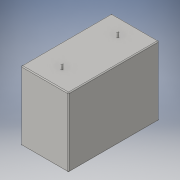
# Autodesk Inventor part: Deep Cycle Battery
Saved by Autodesk Inventor 2016 (Build 200138000, 138)
## iProperties
Created: 2018-07-06
Part Number: Deep Cycle Battery
Material: Generic
Document SubType Name: Modeling
Designer: Kade
Density: 1 g/cm^3
Appearance: Default
Author: Kade
Autodesk Inventor part; units mm, degrees
ref_plane "YZ Plane" through (0, 0, 0) normal (1, 0, 0) x (0, 1, 0)
ref_plane "XZ Plane" through (0, 0, 0) normal (0, 1, 0) x (-1, 0, 0)
ref_plane "XY Plane" through (0, 0, 0) normal (0, 0, 1) x (1, 0, 0)
sketch "Sketch1" plane through (0, 0, 0) normal (0, 1, 0) x (-1, 0, 0)
  line L0 (0, 0) -> (173.228, 0)
  line L1 (173.228, 0) -> (173.228, -330.2)
  line L2 (173.228, -330.2) -> (0, -330.2)
  line L3 (0, -330.2) -> (0, 0)
  dimension "d0" = 173.228
  dimension "d1" = 330.2
  constraints: 8 end point, 2 parallel, 1 horizontal, 1 perpendicular
  measures "d0" distance of L1.end L2.end
  measures "d1" distance of L0.end L1.end
extrude "Extrusion1" add sketch "Sketch1" along normal blind 251.46
fillet "Fillet1" radius 3.175 12 edges at (0, 251.46, -165.1) (-86.614, 251.46, 0) (0, 125.73, 0) (-173.228, 251.46, -165.1) (-86.614, 251.46, -330.2) (0, 125.73, -330.2) (-173.228, 125.73, 0) (-86.614, 0, 0) (0, 0, -165.1) (-173.228, 0, -165.1) (-86.614, 0, -330.2) (-173.228, 125.73, -330.2)
sketch "Sketch2" plane through (0, 251.46, 0) normal (0, 1, 0) x (1, 0, 0)
  circle A0 centre (-86.614, 63.5) radius 3.175
  circle A1 centre (-86.614, 266.7) radius 3.175
  line L0 (0, 3.175) -> (0, 327.025) projected
  line L1 (-173.228, 327.025) -> (-173.228, 3.175) projected
  line L2 (-3.175, 330.2) -> (-170.053, 330.2) projected
  line L3 (-170.053, 0) -> (-3.175, 0) projected
  point P0 (0, 0)
  dimension "d5" = 6.35
  dimension "d6" = 6.35
  dimension "d9" = 86.614
  dimension "d10" = 86.614
  dimension "d11" = 86.614
  dimension "d12" = 63.5
  dimension "d13" = 63.5
  constraints: 2 centre point
  measures "d5" diameter of A0
  measures "d6" diameter of A1
  measures "d9" distance from line of L0 A0.centre
  measures "d10" distance from line of L0 A1.centre
  measures "d11" distance from line of A1.centre L1
  measures "d12" distance from line of L2 A1.centre
  measures "d13" distance from line of L3 A0.centre
extrude "Extrusion2" add sketch "Sketch2" along normal blind 19.05
fillet "Fillet2" radius 3.175 2 edges at (-89.789, 270.51, -63.5) (-89.789, 270.51, -266.7)
equation "\"d10\" = d11"
body "Solid1"
